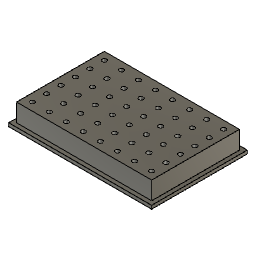
Aluminio v1 (Autodesk Fusion 360 design; units mm, degrees)
Autodesk Fusion 360 part; units mm, degrees
note: some values were not read from the file. Chosen so that the rebuilt part matches the saved one: which face or edge a step refers to.
sketch "Sketch1" plane through (0, 0, 0) normal (0, 0, 1) x (1, 0, 0)
  line L0 (63.88, 42.74) -> (-63.88, 42.74)
  line L1 (-63.88, 42.74) -> (-63.88, -42.74)
  line L2 (-63.88, -42.74) -> (63.88, -42.74)
  line L3 (63.88, -42.74) -> (63.88, 42.74)
  line L4 (63.88, 42.74) -> (-63.88, -42.74) construction
  line L5 (-63.88, 42.74) -> (63.88, -42.74) construction
  dimension "d1" = 127.76
  dimension "d2" = 85.48
  constraint horizontal L0
  constraint perpendicular L0 L1
  constraint parallel L0 L2
  constraint parallel L1 L3
  constraint coincident L4 origin
  constraint coincident L5 origin
  measures "d1" distance of L1.end L2.end
  measures "d2" distance of L0.end L1.end
extrude "Extrude1" add sketch "Sketch1" along normal blind 3
sketch "Sketch2" plane through (0, 0, 3) normal (0, 0, 1) x (-1, 0, 0)
  line L0 (-63.88, 42.74) -> (-63.88, -42.74)
  line L1 (-63.88, -42.74) -> (63.88, -42.74)
  line L2 (63.88, -42.74) -> (63.88, 42.74)
  line L3 (63.88, 42.74) -> (-63.88, 42.74)
  line L4 (60.38, -39.24) -> (-60.38, -39.24)
  line L5 (-60.38, -39.24) -> (-60.38, 39.24)
  line L6 (-60.38, 39.24) -> (60.38, 39.24)
  line L7 (60.38, 39.24) -> (60.38, -39.24)
  line L8 (60.38, -39.24) -> (-60.38, 39.24) construction
  line L9 (-60.38, -39.24) -> (60.38, 39.24) construction
  dimension "d5" = 120.76
  dimension "d6" = 78.48
  constraint horizontal L4
  constraint perpendicular L4 L5
  constraint parallel L4 L6
  constraint parallel L5 L7
  constraint coincident L8 origin
  constraint coincident L9 origin
  measures "d5" distance of L5.end L6.end
  measures "d6" distance of L4.end L5.end
extrude "Extrude2" add sketch "Sketch2" along normal blind 16.05 contours L4 L5 L6 L7
sketch "Sketch3" plane through (0, 0, 0) normal (0, 0, 1) x (1, 0, 0)
sketch "Sketch4" plane through (0, 0, 0) normal (0, 0, 1) x (1, 0, 0)
  line L0 (55.38, 34.24) -> (-55.38, 34.24)
  line L1 (-55.38, 34.24) -> (-55.38, -34.24)
  line L2 (-55.38, -34.24) -> (55.38, -34.24)
  line L3 (55.38, -34.24) -> (55.38, 34.24)
  line L4 (55.38, 34.24) -> (-55.38, -34.24) construction
  line L5 (-55.38, 34.24) -> (55.38, -34.24) construction
  dimension "d9" = 110.76
  dimension "d10" = 68.48
  constraint horizontal L0
  constraint perpendicular L0 L1
  constraint parallel L0 L2
  constraint parallel L1 L3
  constraint coincident L4 origin
  constraint coincident L5 origin
  measures "d9" distance of L1.end L2.end
  measures "d10" distance of L0.end L1.end
sketch "Sketch5" plane through (0, 0, 19.05) normal (0, 0, 1) x (-1, 0, 0)
  line L0 (60.38, 39.24) -> (-60.38, 39.24)
  line L1 (-60.38, 39.24) -> (-60.38, -39.24)
  line L2 (-60.38, -39.24) -> (60.38, -39.24)
  line L3 (60.38, -39.24) -> (60.38, 39.24)
  line L4 (55.38, -34.24) -> (-55.38, -34.24)
  line L5 (-55.38, -34.24) -> (-55.38, 34.24)
  line L6 (-55.38, 34.24) -> (55.38, 34.24)
  line L7 (55.38, 34.24) -> (55.38, -34.24)
  line L8 (55.38, -34.24) -> (-55.38, 34.24) construction
  line L9 (-55.38, -34.24) -> (55.38, 34.24) construction
  dimension "d11" = 110.76
  dimension "d12" = 68.48
  constraint horizontal L4
  constraint perpendicular L4 L5
  constraint parallel L4 L6
  constraint parallel L5 L7
  constraint coincident L8 origin
  constraint coincident L9 origin
  measures "d11" distance of L5.end L6.end
  measures "d12" distance of L4.end L5.end
sketch "Sketch6" plane through (0, 0, 0) normal (0, 0, 1) x (1, 0, 0)
  line L0 (55.38, 34.24) -> (-55.38, 34.24)
  line L1 (-55.38, 34.24) -> (-55.38, -34.24)
sketch "Sketch7" plane through (0, 0, 0) normal (0, 0, 1) x (1, 0, 0)
sketch "Sketch8" plane through (0, 0, 0) normal (0, 0, 1) x (1, 0, 0)
  line L0 (-55.38, 34.24) -> (-55.38, -34.24)
  line L1 (-55.38, -34.24) -> (55.38, -34.24)
  circle A0 centre (-53.38, -32.24) radius 2
  dimension "d15" = 2
  constraint tangent L0 A0
  constraint tangent L1 A0
  measures "d15" radius of A0
sketch "Sketch9" plane through (0, 0, 19.05) normal (0, 0, 1) x (-1, 0, 0)
  line L0 (-55.38, 34.24) -> (55.38, 34.24)
  line L1 (55.38, 34.24) -> (55.38, -34.24)
  circle A0 centre (53.38, 32.24) radius 2
  dimension "d16" = 2
  constraint tangent L0 A0
  constraint tangent L1 A0
  measures "d16" radius of A0
loft "Loft1" cut profiles "Sketch9", "Sketch8" section 1 contours A0 section 2 contours A0
pattern_linear "R-Pattern1" count 8 spacing 15.2429 along (1, 0, 0) count 6 spacing 12.9 along (0, 1, 0) of 1 faces at (-54.9121, -33.5256, 12.7)
